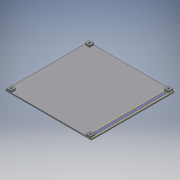
# Autodesk Inventor part: Backplate-housing
Saved by Autodesk Inventor 2016 SP2 (Build 200236200, 236)
## iProperties
Created: 2018-06-21
Part Number: Backplate-housing
Material: Generisch
Document SubType Name: Modeling
Designer: Nils
Density: 1 g/cm^3
Appearance: Vorgabe
Author: Nils
Autodesk Inventor part; units mm, degrees
ref_plane "YZ Plane" through (0, 0, 0) normal (1, 0, 0) x (0, 1, 0)
ref_plane "XZ Plane" through (0, 0, 0) normal (0, 1, 0) x (-1, 0, 0)
ref_plane "XY Plane" through (0, 0, 0) normal (0, 0, 1) x (1, 0, 0)
ref_plane "Arbeitsebene1" through (796.2209, 70.6141, -996.2958) normal (0, 0, -1) x (-1, 0, 0)
sketch "Skizze1" plane through (796.2209, 70.6141, -996.2958) normal (0, 0, -1) x (-1, 0, 0)
  line L0 (-3.9996, -76.75) -> (4.0004, -76.75) construction
  line L1 (-3.9996, 76.75) -> (-3.9996, -76.75) construction
  line L2 (4.0004, 76.75) -> (-3.9996, 76.75) construction
  line L3 (4.0004, 84.25) -> (4.0004, 76.75) construction
  line L4 (-37.8996, 84.25) -> (4.0004, 84.25) construction
  line L5 (-37.8996, 1.75) -> (-37.8996, 84.25) construction
  line L6 (-133.3996, 1.75) -> (-37.8996, 1.75) construction
  line L7 (-133.3996, -84.25) -> (-133.3996, 1.75) construction
  line L8 (4.0004, -84.25) -> (-133.3996, -84.25) construction
  line L9 (4.0004, -76.75) -> (4.0004, -84.25) construction
  line L10 (150.8004, -76.75) -> (142.8004, -76.75) construction
  line L11 (142.8004, -76.75) -> (142.8004, -84.25) construction
  line L12 (142.8004, -84.25) -> (280.2004, -84.25) construction
  line L13 (280.2004, -84.25) -> (280.2004, 1.75) construction
  line L14 (280.2004, 1.75) -> (184.7004, 1.75) construction
  line L15 (184.7004, 1.75) -> (184.7004, 84.25) construction
  line L16 (184.7004, 84.25) -> (142.8004, 84.25) construction
  line L17 (142.8004, 84.25) -> (142.8004, 76.75) construction
  line L18 (142.8004, 76.75) -> (150.8004, 76.75) construction
  line L19 (150.8004, 76.75) -> (150.8004, -76.75) construction
  line L20 (-5.9996, 76.75) -> (-5.9996, -76.75)
  line L21 (152.8004, 76.75) -> (152.8004, -76.75)
  line L22 (-5.9996, 76.75) -> (152.8004, 76.75)
  line L23 (-5.9996, -76.75) -> (152.8004, -76.75)
  point P0 (796.2209, -70.6141)
  constraints: 8 end point, 2 vertical, 1 collinear, 1 parallel, 4 other
extrude "Extrusion1" add sketch "Skizze1" along normal blind 2
sketch "Skizze2" plane through (796.2209, 70.6141, -996.2958) normal (0, 0, 1) x (1, 0, 0)
  line L0 (-152.8004, -76.75) -> (-142.8004, -76.75)
  line L1 (-142.8004, -66.75) -> (-152.8004, -66.75)
  line L2 (-142.8004, -76.75) -> (-142.8004, -66.75)
  line L3 (-152.8004, -66.75) -> (-152.8004, -76.75)
  line L4 (-4.0004, -66.75) -> (5.9996, -66.75)
  line L5 (-4.0004, -76.75) -> (-4.0004, -66.75)
  line L6 (5.9996, -66.75) -> (5.9996, -76.75)
  line L7 (5.9996, -76.75) -> (-4.0004, -76.75)
  line L8 (-152.8004, 66.75) -> (-142.8004, 66.75)
  line L9 (-142.8004, 66.75) -> (-142.8004, 76.75)
  line L10 (-142.8004, 76.75) -> (-152.8004, 76.75)
  line L11 (-152.8004, 76.75) -> (-152.8004, 66.75)
  line L12 (-4.0004, 66.75) -> (-4.0004, 76.75)
  line L13 (5.9996, 66.75) -> (-4.0004, 66.75)
  line L14 (-4.0004, 76.75) -> (5.9996, 76.75)
  line L15 (5.9996, 76.75) -> (5.9996, 66.75)
  point P0 (-796.2209, -70.6141)
  constraints: 32 end point, 8 horizontal, 8 vertical, 16 other
extrude "Extrusion2" add sketch "Skizze2" along normal blind 3.5
sketch "Skizze3" plane through (796.2209, 70.6141, -992.7958) normal (0, 0, 1) x (1, 0, 0)
  circle A0 centre (0.9996, 71.75) radius 1.75
  circle A1 centre (0.9996, -71.75) radius 1.75
  circle A2 centre (-147.8004, 71.75) radius 1.75
  circle A3 centre (-147.8004, -71.75) radius 1.75
  point P0 (-796.2209, -70.6141)
  constraints: 4 centre point, 8 other
extrude "Extrusion3" cut sketch "Skizze3" against normal blind 15.5
sketch "Skizze4" plane through (796.2209, 70.6141, -998.2958) normal (0, 0, -1) x (-1, 0, 0)
  circle A0 centre (-0.9996, 71.75) radius 1.75 projected
  circle A1 centre (-0.9996, 71.75) radius 3
  circle A2 centre (-0.9996, -71.75) radius 1.75 projected
  circle A3 centre (147.8004, -71.75) radius 1.75 projected
  circle A4 centre (147.8004, 71.75) radius 1.75 projected
  circle A5 centre (147.8004, 71.75) radius 1.75 projected
  circle A6 centre (147.8004, 71.75) radius 3
  circle A7 centre (-0.9996, -71.75) radius 1.75 projected
  circle A8 centre (-0.9996, -71.75) radius 3
  circle A9 centre (147.8004, -71.75) radius 1.75 projected
  circle A10 centre (147.8004, -71.75) radius 3
  point P0 (796.2209, -70.6141)
  dimension "d20" = 6
  dimension "d21" = 6
  dimension "d22" = 6
  dimension "d23" = 6
  constraints: 4 centre point, 4 coincident
  measures "d20" diameter of A1
  measures "d21" diameter of A8
  measures "d22" diameter of A10
  measures "d23" diameter of A6
extrude "Extrusion4" cut sketch "Skizze4" against normal blind 3.4
equation "\"d21\" = d20"
equation "\"d22\" = d21"
equation "\"d23\" = d21"
